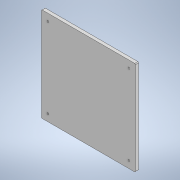
# Autodesk Inventor part: Etage
Saved by Autodesk Inventor 2020.2 (Build 242310000, 310)
## iProperties
Created: 2020-01-21
Part Number: Etage
Material: Générique
Document SubType Name: Modeling
Designer: anton
Density: 1 g/cm^3
Appearance: Par défaut
Author: anton
Autodesk Inventor part; units mm, degrees
ref_plane "YZ Plane" through (0, 0, 0) normal (1, 0, 0) x (0, 1, 0)
ref_plane "XZ Plane" through (0, 0, 0) normal (0, 1, 0) x (-1, 0, 0)
ref_plane "XY Plane" through (0, 0, 0) normal (0, 0, 1) x (1, 0, 0)
sketch "Esquisse1" plane through (0, 0, 0) normal (0, 0, 1) x (1, 0, 0)
  line L0 (-42.4556, 24.926) -> (137.5444, 24.926)
  line L1 (137.5444, 24.926) -> (137.5444, -155.074)
  line L2 (137.5444, -155.074) -> (-42.4556, -155.074)
  line L3 (-42.4556, -155.074) -> (-42.4556, 24.926)
  point P0 (0, 0)
  dimension "d0" = 180
  dimension "d1" = 180
  constraints: 8 end point, 2 parallel, 1 horizontal, 1 perpendicular
  measures "d0" distance of L0.start L0.end
  measures "d1" distance of L2.end L0.start
extrude "Extrusion1" add sketch "Esquisse1" along normal blind 6
sketch "Esquisse2" plane through (0, 0, 6) normal (0, 0, 1) x (1, 0, 0)
  circle A0 centre (-29.9556, 11.426) radius 2.2339
  circle A1 centre (125.0444, 11.426) radius 4.5426
  circle A2 centre (125.0444, -141.574) radius 4.8644
  circle A3 centre (-29.9556, -141.574) radius 7.3197
  line L0 (-42.4556, 24.926) -> (-42.4556, -155.074) projected
  line L1 (-42.4556, -155.074) -> (137.5444, -155.074) projected
  line L2 (137.5444, -155.074) -> (137.5444, 24.926) projected
  line L3 (137.5444, 24.926) -> (-42.4556, 24.926) projected
  point P0 (0, 0)
  dimension "d19" = 153
  dimension "d20" = 155
  dimension "d21" = 153
  dimension "d22" = 155
  dimension "d25" = 12.5
  dimension "d26" = 12.5
  dimension "d27" = 13.5
  dimension "d28" = 13.5
  constraints: 4 centre point
  measures "d19" distance of A2.centre A1.centre
  measures "d20" distance of A3.centre A2.centre
  measures "d21" distance of A0.centre A3.centre
  measures "d22" distance of A1.centre A0.centre
  measures "d25" distance from line of L0 A0.centre
  measures "d26" distance from line of L0 A3.centre
  measures "d27" distance from line of L3 A0.centre
  measures "d28" distance from line of L1 A2.centre
hole "Perçage1" at (-29.9556, 11.426, 6) at (125.0444, 11.426, 6) at (125.0444, -141.574, 6) at (-29.9556, -141.574, 6) direction (0, 0, -1) diameter 3.5 end through all
fillet "Congé2" radius 1.5 4 edges at (-42.4556, 24.926, 3) (137.5444, 24.926, 3) (137.5444, -155.074, 3) (-42.4556, -155.074, 3)
